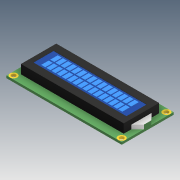
# Autodesk Inventor part: lcd-16x2-display
Saved by Autodesk Inventor 2017 (Build 210142000, 142)
## iProperties
Created: 2018-07-15
Part Number: lcd-16x2-display
Material: Generic
Document SubType Name: Modeling
Designer: Luiz Gustavo
Density: 1 g/cm^3
Appearance: Steel Blue
Author: Luiz Gustavo
Autodesk Inventor part; units mm, degrees
ref_plane "YZ Plane" through (0, 0, 0) normal (1, 0, 0) x (0, 1, 0)
ref_plane "XZ Plane" through (0, 0, 0) normal (0, 1, 0) x (-1, 0, 0)
ref_plane "XY Plane" through (0, 0, 0) normal (0, 0, 1) x (1, 0, 0)
sketch "Sketch1" plane through (0, 0, 0) normal (0, 0, 1) x (1, 0, 0)
  line L0 (-40, 18) -> (40, 18)
  line L1 (40, 18) -> (40, -18)
  line L2 (40, -18) -> (-40, -18)
  line L3 (-40, -18) -> (-40, 18)
  line L4 (-40, 18) -> (40, -18) construction
  line L5 (40, 18) -> (-40, -18) construction
  line L6 (-37.5, -15.5) -> (37.5, -15.5) construction
  line L7 (37.5, -15.5) -> (37.5, 15.5) construction
  line L8 (37.5, 15.5) -> (-37.5, 15.5) construction
  line L9 (-37.5, 15.5) -> (-37.5, -15.5) construction
  line L10 (-37.5, -15.5) -> (37.5, 15.5) construction
  line L11 (37.5, -15.5) -> (-37.5, 15.5) construction
  circle A0 centre (-37.5, 15.5) radius 1.5
  circle A1 centre (37.5, 15.5) radius 1.5
  circle A2 centre (37.5, -15.5) radius 1.5
  circle A3 centre (-37.5, -15.5) radius 1.5
  circle A4 centre (-37.5, 15.5) radius 2.5
  circle A5 centre (37.5, 15.5) radius 2.5
  circle A6 centre (37.5, -15.5) radius 2.5
  circle A7 centre (-37.5, -15.5) radius 2.5
  point P0 (0, 0)
  dimension "d0" = 80
  dimension "d1" = 36
  dimension "d2" = 75
  dimension "d3" = 31
  dimension "d4" = 3
  dimension "d5" = 5
  constraints: 24 end point, 8 centre point, 8 coincident, 6 equal radius, 4 midpoint, 4 parallel, 2 horizontal, 2 perpendicular
  measures "d0" distance of L0.start L0.end
  measures "d1" distance of L2.end L0.start
  measures "d2" distance of L7.end L8.end
  measures "d3" distance of L8.end L6.start
  measures "d4" diameter of A0
  measures "d5" diameter of A4
extrude "Extrusion1" add sketch "Sketch1" along normal mid plane 1.6 contours L0 A4 L3 | L0 A5 L1 A6 L2 A7 L3 A4 | L0 L1 A5 | A7 L2 L3 | L1 L2 A6
extrude "Extrusion2" add sketch "Sketch1" along normal mid plane 1.65 contours A4 | A5 | A7 | A6
sketch "Sketch2" plane through (0, 0, 0) normal (0, 0, 1) x (1, 0, 0)
  line L0 (-35.65, 12.25) -> (35.65, 12.25)
  line L1 (35.65, 12.25) -> (35.65, -12.25)
  line L2 (35.65, -12.25) -> (-35.65, -12.25)
  line L3 (-35.65, -12.25) -> (-35.65, 12.25)
  line L4 (-35.65, 12.25) -> (35.65, -12.25) construction
  line L5 (35.65, 12.25) -> (-35.65, -12.25) construction
  line L6 (-32.25, -7) -> (32.25, -7)
  line L7 (32.25, -7) -> (32.25, 7)
  line L8 (32.25, 7) -> (-32.25, 7)
  line L9 (-32.25, 7) -> (-32.25, -7)
  line L10 (-32.25, -7) -> (32.25, 7) construction
  line L11 (32.25, -7) -> (-32.25, 7) construction
  point P0 (0, 0)
  dimension "d10" = 24.5
  dimension "d11" = 71.3
  dimension "d12" = 64.5
  dimension "d13" = 14
  constraints: 24 end point, 4 midpoint, 4 parallel, 2 horizontal, 2 perpendicular
  measures "d10" distance of L2.end L0.start
  measures "d11" distance of L0.start L0.end
  measures "d12" distance of L8.end L7.end
  measures "d13" distance of L7.end L6.end
extrude "Extrusion3" add sketch "Sketch2" along normal blind 7
extrude "Extrusion4" add sketch "Sketch2" along normal blind 6.9 contours L9 L8 L7 L6
sketch "Sketch3" plane through (0, 0, 0) normal (0, 0, 1) x (1, 0, 0)
  circle A0 centre (-30, 15.46) radius 0.5
  line L0 (-40, 18) -> (40, 18) construction
  line L1 (-31, 15.46) -> (-31, 18)
  line L2 (-31, 18) -> (-29, 18)
  line L3 (-29, 18) -> (-29, 15.46)
  arc A1 (-31, 15.46) -> (-29, 15.46) centre (-30, 15.46) ccw
  arc A2 (-28.46, 15.46) -> (-26.46, 15.46) centre (-27.46, 15.46) ccw
  line L4 (-28.46, 15.46) -> (-28.46, 18)
  line L5 (-28.46, 18) -> (-26.46, 18)
  line L6 (-26.46, 18) -> (-26.46, 15.46)
  circle A3 centre (-27.46, 15.46) radius 0.5
  arc A4 (-25.92, 15.46) -> (-23.92, 15.46) centre (-24.92, 15.46) ccw
  line L7 (-25.92, 15.46) -> (-25.92, 18)
  line L8 (-25.92, 18) -> (-23.92, 18)
  line L9 (-23.92, 18) -> (-23.92, 15.46)
  circle A5 centre (-24.92, 15.46) radius 0.5
  arc A6 (-23.38, 15.46) -> (-21.38, 15.46) centre (-22.38, 15.46) ccw
  line L10 (-23.38, 15.46) -> (-23.38, 18)
  line L11 (-23.38, 18) -> (-21.38, 18)
  line L12 (-21.38, 18) -> (-21.38, 15.46)
  circle A7 centre (-22.38, 15.46) radius 0.5
  arc A8 (-20.84, 15.46) -> (-18.84, 15.46) centre (-19.84, 15.46) ccw
  line L13 (-20.84, 15.46) -> (-20.84, 18)
  line L14 (-20.84, 18) -> (-18.84, 18)
  line L15 (-18.84, 18) -> (-18.84, 15.46)
  circle A9 centre (-19.84, 15.46) radius 0.5
  arc A10 (-18.3, 15.46) -> (-16.3, 15.46) centre (-17.3, 15.46) ccw
  line L16 (-18.3, 15.46) -> (-18.3, 18)
  line L17 (-18.3, 18) -> (-16.3, 18)
  line L18 (-16.3, 18) -> (-16.3, 15.46)
  circle A11 centre (-17.3, 15.46) radius 0.5
  arc A12 (-15.76, 15.46) -> (-13.76, 15.46) centre (-14.76, 15.46) ccw
  line L19 (-15.76, 15.46) -> (-15.76, 18)
  line L20 (-15.76, 18) -> (-13.76, 18)
  line L21 (-13.76, 18) -> (-13.76, 15.46)
  circle A13 centre (-14.76, 15.46) radius 0.5
  arc A14 (-13.22, 15.46) -> (-11.22, 15.46) centre (-12.22, 15.46) ccw
  line L22 (-13.22, 15.46) -> (-13.22, 18)
  line L23 (-13.22, 18) -> (-11.22, 18)
  line L24 (-11.22, 18) -> (-11.22, 15.46)
  circle A15 centre (-12.22, 15.46) radius 0.5
  arc A16 (-10.68, 15.46) -> (-8.68, 15.46) centre (-9.68, 15.46) ccw
  line L25 (-10.68, 15.46) -> (-10.68, 18)
  line L26 (-10.68, 18) -> (-8.68, 18)
  line L27 (-8.68, 18) -> (-8.68, 15.46)
  circle A17 centre (-9.68, 15.46) radius 0.5
  arc A18 (-8.14, 15.46) -> (-6.14, 15.46) centre (-7.14, 15.46) ccw
  line L28 (-8.14, 15.46) -> (-8.14, 18)
  line L29 (-8.14, 18) -> (-6.14, 18)
  line L30 (-6.14, 18) -> (-6.14, 15.46)
  circle A19 centre (-7.14, 15.46) radius 0.5
  arc A20 (-5.6, 15.46) -> (-3.6, 15.46) centre (-4.6, 15.46) ccw
  line L31 (-5.6, 15.46) -> (-5.6, 18)
  line L32 (-5.6, 18) -> (-3.6, 18)
  line L33 (-3.6, 18) -> (-3.6, 15.46)
  circle A21 centre (-4.6, 15.46) radius 0.5
  arc A22 (-3.06, 15.46) -> (-1.06, 15.46) centre (-2.06, 15.46) ccw
  line L34 (-3.06, 15.46) -> (-3.06, 18)
  line L35 (-3.06, 18) -> (-1.06, 18)
  line L36 (-1.06, 18) -> (-1.06, 15.46)
  circle A23 centre (-2.06, 15.46) radius 0.5
  arc A24 (-0.52, 15.46) -> (1.48, 15.46) centre (0.48, 15.46) ccw
  line L37 (-0.52, 15.46) -> (-0.52, 18)
  line L38 (-0.52, 18) -> (1.48, 18)
  line L39 (1.48, 18) -> (1.48, 15.46)
  circle A25 centre (0.48, 15.46) radius 0.5
  arc A26 (2.02, 15.46) -> (4.02, 15.46) centre (3.02, 15.46) ccw
  line L40 (2.02, 15.46) -> (2.02, 18)
  line L41 (2.02, 18) -> (4.02, 18)
  line L42 (4.02, 18) -> (4.02, 15.46)
  circle A27 centre (3.02, 15.46) radius 0.5
  arc A28 (4.56, 15.46) -> (6.56, 15.46) centre (5.56, 15.46) ccw
  line L43 (4.56, 15.46) -> (4.56, 18)
  line L44 (4.56, 18) -> (6.56, 18)
  line L45 (6.56, 18) -> (6.56, 15.46)
  circle A29 centre (5.56, 15.46) radius 0.5
  arc A30 (7.1, 15.46) -> (9.1, 15.46) centre (8.1, 15.46) ccw
  line L46 (7.1, 15.46) -> (7.1, 18)
  line L47 (7.1, 18) -> (9.1, 18)
  line L48 (9.1, 18) -> (9.1, 15.46)
  circle A31 centre (8.1, 15.46) radius 0.5
  point P0 (0, 0)
  dimension "d18" = 1
  dimension "d19" = 2.54
  dimension "d20" = 2
  dimension "d21" = 10
  dimension "d24" = 2.54
  constraints: 96 end point, 32 centre point, 32 point on circle, 16 coincident, 3 perpendicular, 2 tangent, 1 collinear, 1 horizontal, 165 other
  measures "d18" diameter of A0
  measures "d19" distance from line of A0.centre L0
  measures "d20" distance between parallel lines of L3 L1
  measures "d21" horizontal distance of A0.centre L0.start
  measures "d24" distance of A1.centre A2.centre
extrude "Extrusion5" add sketch "Sketch3" along normal mid plane 1.65
extrude "Extrusion6" cut sketch "Sketch3" against normal through all contours A0 | A3 | A5 | A7 | A9 | A11 | A13 | A15 | A17 | A19 | A21 | A23 | A25 | A27 | A29 | L46 L47 L48 A30
sketch "Sketch4" plane through (0, 0, 6.9) normal (0, 0, 1) x (1, 0, 0)
  line L0 (32.25, -7) -> (-32.25, -7) projected
  line L1 (32.25, 7) -> (32.25, -7) projected
  line L2 (-32.25, 7) -> (32.25, 7) projected
  line L3 (-32.25, -7) -> (-32.25, 7) projected
  line L4 (-28.1, 5.75) -> (-25.3, 5.75)
  line L5 (-25.3, 5.75) -> (-25.3, 0.5)
  line L6 (-25.3, 0.5) -> (-28.1, 0.5)
  line L7 (-28.1, 0.5) -> (-28.1, 5.75)
  line L8 (-28.1, 5.75) -> (-25.3, 0.5) construction
  line L9 (-25.3, 5.75) -> (-28.1, 0.5) construction
  line L10 (-32.25, -7) -> (-32.25, 7) construction
  line L11 (-32.25, 0) -> (32.25, 0) construction
  line L12 (-28.1, -5.75) -> (-25.3, -5.75)
  line L13 (-25.3, -5.75) -> (-25.3, -0.5)
  line L14 (-25.3, -0.5) -> (-28.1, -0.5)
  line L15 (-28.1, -0.5) -> (-28.1, -5.75)
  line L16 (-28.1, -5.75) -> (-25.3, -0.5) construction
  line L17 (-25.3, -5.75) -> (-28.1, -0.5) construction
  line L18 (-21.74, 5.75) -> (-21.74, 0.5)
  line L19 (-24.54, 5.75) -> (-21.74, 5.75)
  line L20 (-24.54, 0.5) -> (-24.54, 5.75)
  line L21 (-21.74, 0.5) -> (-24.54, 0.5)
  line L22 (-21.74, -5.75) -> (-21.74, -0.5)
  line L23 (-21.74, -0.5) -> (-24.54, -0.5)
  line L24 (-24.54, -5.75) -> (-21.74, -5.75)
  line L25 (-24.54, -0.5) -> (-24.54, -5.75)
  line L26 (-18.18, 5.75) -> (-18.18, 0.5)
  line L27 (-20.98, 5.75) -> (-18.18, 5.75)
  line L28 (-20.98, 0.5) -> (-20.98, 5.75)
  line L29 (-18.18, 0.5) -> (-20.98, 0.5)
  line L30 (-18.18, -5.75) -> (-18.18, -0.5)
  line L31 (-18.18, -0.5) -> (-20.98, -0.5)
  line L32 (-20.98, -5.75) -> (-18.18, -5.75)
  line L33 (-20.98, -0.5) -> (-20.98, -5.75)
  line L34 (-14.62, 5.75) -> (-14.62, 0.5)
  line L35 (-17.42, 5.75) -> (-14.62, 5.75)
  line L36 (-17.42, 0.5) -> (-17.42, 5.75)
  line L37 (-14.62, 0.5) -> (-17.42, 0.5)
  line L38 (-14.62, -5.75) -> (-14.62, -0.5)
  line L39 (-14.62, -0.5) -> (-17.42, -0.5)
  line L40 (-17.42, -5.75) -> (-14.62, -5.75)
  line L41 (-17.42, -0.5) -> (-17.42, -5.75)
  line L42 (-11.06, 5.75) -> (-11.06, 0.5)
  line L43 (-13.86, 5.75) -> (-11.06, 5.75)
  line L44 (-13.86, 0.5) -> (-13.86, 5.75)
  line L45 (-11.06, 0.5) -> (-13.86, 0.5)
  line L46 (-11.06, -5.75) -> (-11.06, -0.5)
  line L47 (-11.06, -0.5) -> (-13.86, -0.5)
  line L48 (-13.86, -5.75) -> (-11.06, -5.75)
  line L49 (-13.86, -0.5) -> (-13.86, -5.75)
  line L50 (-7.5, 5.75) -> (-7.5, 0.5)
  line L51 (-10.3, 5.75) -> (-7.5, 5.75)
  line L52 (-10.3, 0.5) -> (-10.3, 5.75)
  line L53 (-7.5, 0.5) -> (-10.3, 0.5)
  line L54 (-7.5, -5.75) -> (-7.5, -0.5)
  line L55 (-7.5, -0.5) -> (-10.3, -0.5)
  line L56 (-10.3, -5.75) -> (-7.5, -5.75)
  line L57 (-10.3, -0.5) -> (-10.3, -5.75)
  line L58 (-3.94, 5.75) -> (-3.94, 0.5)
  line L59 (-6.74, 5.75) -> (-3.94, 5.75)
  line L60 (-6.74, 0.5) -> (-6.74, 5.75)
  line L61 (-3.94, 0.5) -> (-6.74, 0.5)
  line L62 (-3.94, -5.75) -> (-3.94, -0.5)
  line L63 (-3.94, -0.5) -> (-6.74, -0.5)
  line L64 (-6.74, -5.75) -> (-3.94, -5.75)
  line L65 (-6.74, -0.5) -> (-6.74, -5.75)
  line L66 (-0.38, 5.75) -> (-0.38, 0.5)
  line L67 (-3.18, 5.75) -> (-0.38, 5.75)
  line L68 (-3.18, 0.5) -> (-3.18, 5.75)
  line L69 (-0.38, 0.5) -> (-3.18, 0.5)
  line L70 (-0.38, -5.75) -> (-0.38, -0.5)
  line L71 (-0.38, -0.5) -> (-3.18, -0.5)
  line L72 (-3.18, -5.75) -> (-0.38, -5.75)
  line L73 (-3.18, -0.5) -> (-3.18, -5.75)
  line L74 (3.18, 5.75) -> (3.18, 0.5)
  line L75 (0.38, 5.75) -> (3.18, 5.75)
  line L76 (0.38, 0.5) -> (0.38, 5.75)
  line L77 (3.18, 0.5) -> (0.38, 0.5)
  line L78 (3.18, -5.75) -> (3.18, -0.5)
  line L79 (3.18, -0.5) -> (0.38, -0.5)
  line L80 (0.38, -5.75) -> (3.18, -5.75)
  line L81 (0.38, -0.5) -> (0.38, -5.75)
  line L82 (6.74, 5.75) -> (6.74, 0.5)
  line L83 (3.94, 5.75) -> (6.74, 5.75)
  line L84 (3.94, 0.5) -> (3.94, 5.75)
  line L85 (6.74, 0.5) -> (3.94, 0.5)
  line L86 (6.74, -5.75) -> (6.74, -0.5)
  line L87 (6.74, -0.5) -> (3.94, -0.5)
  line L88 (3.94, -5.75) -> (6.74, -5.75)
  line L89 (3.94, -0.5) -> (3.94, -5.75)
  line L90 (10.3, 5.75) -> (10.3, 0.5)
  line L91 (7.5, 5.75) -> (10.3, 5.75)
  line L92 (7.5, 0.5) -> (7.5, 5.75)
  line L93 (10.3, 0.5) -> (7.5, 0.5)
  line L94 (10.3, -5.75) -> (10.3, -0.5)
  line L95 (10.3, -0.5) -> (7.5, -0.5)
  line L96 (7.5, -5.75) -> (10.3, -5.75)
  line L97 (7.5, -0.5) -> (7.5, -5.75)
  line L98 (13.86, 5.75) -> (13.86, 0.5)
  line L99 (11.06, 5.75) -> (13.86, 5.75)
  line L100 (11.06, 0.5) -> (11.06, 5.75)
  line L101 (13.86, 0.5) -> (11.06, 0.5)
  line L102 (13.86, -5.75) -> (13.86, -0.5)
  line L103 (13.86, -0.5) -> (11.06, -0.5)
  line L104 (11.06, -5.75) -> (13.86, -5.75)
  line L105 (11.06, -0.5) -> (11.06, -5.75)
  line L106 (17.42, 5.75) -> (17.42, 0.5)
  line L107 (14.62, 5.75) -> (17.42, 5.75)
  line L108 (14.62, 0.5) -> (14.62, 5.75)
  line L109 (17.42, 0.5) -> (14.62, 0.5)
  line L110 (17.42, -5.75) -> (17.42, -0.5)
  line L111 (17.42, -0.5) -> (14.62, -0.5)
  line L112 (14.62, -5.75) -> (17.42, -5.75)
  line L113 (14.62, -0.5) -> (14.62, -5.75)
  line L114 (20.98, 5.75) -> (20.98, 0.5)
  line L115 (18.18, 5.75) -> (20.98, 5.75)
  line L116 (18.18, 0.5) -> (18.18, 5.75)
  line L117 (20.98, 0.5) -> (18.18, 0.5)
  line L118 (20.98, -5.75) -> (20.98, -0.5)
  line L119 (20.98, -0.5) -> (18.18, -0.5)
  line L120 (18.18, -5.75) -> (20.98, -5.75)
  line L121 (18.18, -0.5) -> (18.18, -5.75)
  line L122 (24.54, 5.75) -> (24.54, 0.5)
  line L123 (21.74, 5.75) -> (24.54, 5.75)
  line L124 (21.74, 0.5) -> (21.74, 5.75)
  line L125 (24.54, 0.5) -> (21.74, 0.5)
  line L126 (24.54, -5.75) -> (24.54, -0.5)
  line L127 (24.54, -0.5) -> (21.74, -0.5)
  line L128 (21.74, -5.75) -> (24.54, -5.75)
  line L129 (21.74, -0.5) -> (21.74, -5.75)
  line L130 (28.1, 5.75) -> (28.1, 0.5)
  line L131 (25.3, 5.75) -> (28.1, 5.75)
  line L132 (25.3, 0.5) -> (25.3, 5.75)
  line L133 (28.1, 0.5) -> (25.3, 0.5)
  line L134 (28.1, -5.75) -> (28.1, -0.5)
  line L135 (28.1, -0.5) -> (25.3, -0.5)
  line L136 (25.3, -5.75) -> (28.1, -5.75)
  line L137 (25.3, -0.5) -> (25.3, -5.75)
  point P0 (0, 0)
  point P1 (-26.7, 3.125)
  point P2 (-26.7, -3.125)
  dimension "d34" = 11.5
  dimension "d35" = 4.15
  dimension "d38" = 3.56
  dimension "d43" = 1
  dimension "d44" = 2.8
  dimension "d45" = 4.15
  constraints: 266 end point, 6 midpoint, 5 symmetric about line, 2 horizontal, 2 parallel, 1 perpendicular, 240 other
  measures "d34" distance between parallel lines of L12 L4
  measures "d35" distance between parallel lines of L3 L7
  measures "d38" distance of L4.end L18.start
  measures "d43" distance between parallel lines of L14 L6
  measures "d44" distance of L4.start L4.end
  measures "d45" distance between parallel lines of L1 L130
extrude "Extrusion7" add sketch "Sketch4" along normal blind 0.1 contours L4 L5 L6 L7 | L15 L14 L13 L12 | L18 L21 L20 L19 | L24 L25 L23 L22 | L26 L29 L28 L27 | L32 L33 L31 L30 | L34 L37 L36 L35 | L40 L41 L39 L38 | L42 L45 L44 L43 | L48 L49 L47 L46 | L50 L53 L52 L51 | L56 L57 L55 L54 | L58 L61 L60 L59 | L64 L65 L63 L62 | L66 L69 L68 L67 | L72 L73 L71 L70 | L74 L77 L76 L75 | L80 L81 L79 L78 | L82 L85 L84 L83 | L88 L89 L87 L86 | L90 L93 L92 L91 | L96 L97 L95 L94 | L98 L101 L100 L99 | L104 L105 L103 L102 | L106 L109 L108 L107 | L112 L113 L111 L110 | L114 L117 L116 L115 | L120 L121 L119 L118 | L122 L125 L124 L123 | L128 L129 L127 L126 | L130 L133 L132 L131 | L136 L137 L135 L134
sketch "Sketch5" plane through (0, 0, 0.8) normal (0, 0, 1) x (1, 0, 0)
  line L0 (35.65, -12.25) -> (35.65, 12.25) projected
  line L1 (40, -15.5) -> (40, 15.5) projected
  line L2 (35.65, 7) -> (40, 2.5)
  line L3 (40, -2.5) -> (35.65, -7)
  line L4 (35.65, 0) -> (40, 0) construction
  point P0 (0, 0)
  dimension "d48" = 5
  dimension "d49" = 14
  constraints: 6 end point, 4 point on line, 2 midpoint, 1 other
  measures "d48" distance of L3.start L2.end
  measures "d49" distance of L3.end L2.start
extrude "Extrusion8" add sketch "Sketch5" along normal blind 2.8
body "Solid1"
